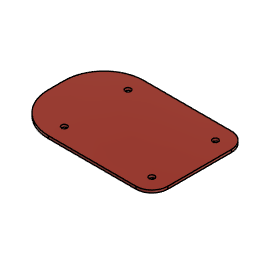
comp207 micro mouse pcb basic layout (Autodesk Fusion 360 design; units mm, degrees)
Autodesk Fusion 360 part; units mm, degrees
note: some values were not read from the file. Set by a fixed rule: which sketch regions a step uses.
sketch "Sketch4" plane through (0, 0, 0) normal (0, 0, 1) x (1, 0, 0)
  line L0 (0, 0) -> (90, 0)
  line L1 (90, 0) -> (90, -60)
  line L2 (90, -60) -> (0, -60)
  line L3 (0, -60) -> (0, 0)
  dimension "d13" = 90
  dimension "d14" = 60
  constraint horizontal L0
  constraint vertical L1
  constraint horizontal L2
  constraint vertical L3
  constraint coincident L0.start L3.end
  measures "d13" distance of L0.start L0.end
  measures "d14" distance of L0.start L2.end
extrude "Extrude3" add sketch "Sketch4" along normal blind 1.6
fillet "Fillet1" radius 25 2 edges at (0, -60, 0.8) (0, 0, 0.8)
fillet "Fillet2" radius 10 2 edges at (90, -60, 0.8) (90, 0, 0.8)
sketch "Sketch5" plane through (0, 0, 1.6) normal (0, 0, 1) x (-1, 0, 0)
  arc A0 (-90, 10) -> (-80, 0) centre (-80, 10) ccw
  line L0 (-80, 0) -> (-25, 0)
  arc A1 (-25, 0) -> (0, 25) centre (-25, 25) ccw
  line L1 (0, 25) -> (0, 35)
  arc A2 (0, 35) -> (-25, 60) centre (-25, 35) ccw
  line L2 (-25, 60) -> (-80, 60)
  arc A3 (-80, 60) -> (-90, 50) centre (-80, 50) ccw
  line L3 (-90, 50) -> (-90, 10)
  line L4 (-80, 10) -> (-25, 10)
  line L5 (-25, 10) -> (-25, 50)
  line L6 (-25, 50) -> (-80, 50)
  line L7 (-80, 50) -> (-80, 10)
  circle A4 centre (-80, 10) radius 1.75
  circle A5 centre (-25, 10) radius 1.75
  circle A6 centre (-25, 50) radius 1.75
  circle A7 centre (-80, 50) radius 1.75
  dimension "d21" = 3.5
  dimension "d22" = 3.5
  dimension "d23" = 3.5
  dimension "d24" = 3.5
  constraint horizontal L4
  constraint vertical L5
  constraint horizontal L6
  constraint vertical L7
  constraint coincident A0.centre L4.start
  constraint coincident L4.end L5.start
  constraint coincident L5.end L6.start
  constraint coincident A3.centre L6.end
  measures "d21" diameter of A4
  measures "d22" diameter of A5
  measures "d23" diameter of A6
  measures "d24" diameter of A7
extrude "Extrude4" cut sketch "Sketch5" against normal blind 2 contours L4 L7 A4 | L4 L7 A4 | L4 L5 A5 | L4 L5 A5 | L6 L7 A7 | L6 L7 A7 | L5 L6 A6 | L5 L6 A6
sketch "Sketch6" plane through (0, 0, 1.6) normal (0, 0, 1) x (-1, 0, 0)
  circle A0 centre (-80, 10) radius 1.75
  circle A1 centre (-80, 50) radius 1.75
  circle A2 centre (-25, 10) radius 1.75
  circle A3 centre (-25, 50) radius 1.75
  arc A4 (-90, 10) -> (-80, 0) centre (-80, 10) ccw
  line L0 (-80, 0) -> (-25, 0)
  arc A5 (-25, 0) -> (0, 25) centre (-25, 25) ccw
  line L1 (0, 25) -> (0, 35)
  arc A6 (0, 35) -> (-25, 60) centre (-25, 35) ccw
  line L2 (-25, 60) -> (-80, 60)
  arc A7 (-80, 60) -> (-90, 50) centre (-80, 50) ccw
  line L3 (-90, 50) -> (-90, 10)
sketch "Sketch7" plane through (0, 0, 1.6) normal (0, 0, 1) x (-1, 0, 0)
  circle A0 centre (-80, 10) radius 1.75
  circle A1 centre (-80, 50) radius 1.75
  circle A2 centre (-25, 10) radius 1.75
  circle A3 centre (-25, 50) radius 1.75
  arc A4 (-90, 10) -> (-80, 0) centre (-80, 10) ccw
  line L0 (-80, 0) -> (-25, 0)
  arc A5 (-25, 0) -> (0, 25) centre (-25, 25) ccw
  line L1 (0, 25) -> (0, 35)
  arc A6 (0, 35) -> (-25, 60) centre (-25, 35) ccw
  line L2 (-25, 60) -> (-80, 60)
  arc A7 (-80, 60) -> (-90, 50) centre (-80, 50) ccw
  line L3 (-90, 50) -> (-90, 10)
